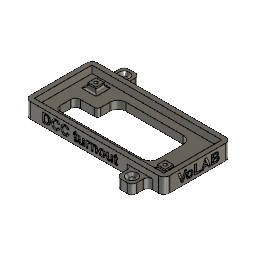
supportCarteDecodeurAiguillage_v4 (Autodesk Fusion 360 design; units mm, degrees)
Autodesk Fusion 360 part; units mm, degrees
note: some values were not read from the file. Chosen so that the rebuilt part matches the saved one: the layout of a text. Set by a fixed rule: which sketch regions a step uses.
sketch "Sketch1" plane through (0, 0, 0) normal (0, 0, 1) x (1, 0, 0)
  line L0 (38.5, -15.24) -> (-38.5, -15.24)
  line L1 (-38.5, -15.24) -> (-38.5, 15.24)
  line L2 (-38.5, 15.24) -> (38.5, 15.24)
  line L3 (38.5, 15.24) -> (38.5, -15.24)
  line L4 (38.5, -15.24) -> (-38.5, 15.24) construction
  line L5 (-38.5, -15.24) -> (38.5, 15.24) construction
  dimension "d1" = 77
  dimension "d2" = 30.48
extrude "Extrude1" add sketch "Sketch1" along normal blind 1.6 makes body 1
sketch "Sketch2" plane through (0, 0, 1.6) normal (0, 0, 1) x (-1, 0, 0)
  line L0 (-38.5, -15.24) -> (38.5, -15.24)
  line L1 (38.5, -15.24) -> (38.5, 15.24)
  line L2 (38.5, 15.24) -> (-38.5, 15.24)
  line L3 (-38.5, 15.24) -> (-38.5, -15.24)
  circle A0 centre (-34.69, 11.43) radius 1.75
  circle A1 centre (31.35, -11.43) radius 1.75
  dimension "d5" = 22.86
  dimension "d6" = 3.5
  dimension "d7" = 3.81
  dimension "d8" = 3.81
  dimension "d9" = 66.04
  dimension "d10" = 4.33
  measures "d6" diameter of A0
extrude "Extrude2" cut sketch "Sketch2" against normal through all contours A0 | A1 bodies 1
copy_body "Body->Comp1" bodies 1 removing the originals makes body 2 in component "carte"
sketch "Sketch3" plane through (0, 0, 0) normal (0, 0, 1) x (1, 0, 0)
  line L0 (43.5, -21) -> (-43.5, -21)
  line L1 (-43.5, -21) -> (-43.5, 21)
  line L2 (-43.5, 21) -> (43.5, 21)
  line L3 (43.5, 21) -> (43.5, -21)
  line L4 (43.5, -21) -> (-43.5, 21) construction
  line L5 (-43.5, -21) -> (43.5, 21) construction
  dimension "d12" = 87
  dimension "d13" = 42
extrude "Extrude3" add sketch "Sketch3" against normal blind 5 from surface at -3 separate body makes body 3
sketch "Sketch4" plane through (0, 0, -3) normal (0, 0, 1) x (-1, 0, 0)
  line L0 (-43.5, -21) -> (43.5, -21)
  line L1 (43.5, -21) -> (43.5, 21)
  line L2 (43.5, 21) -> (-43.5, 21)
  line L3 (-43.5, 21) -> (-43.5, -21)
  circle A0 centre (-34.69, 11.43) radius 1.75
  circle A1 centre (31.35, -11.43) radius 1.75
  line L4 (-37.23, 13.97) -> (-32.15, 13.97)
  line L5 (-32.15, 13.97) -> (-32.15, 8.89)
  line L6 (-32.15, 8.89) -> (-37.23, 8.89)
  line L7 (-37.23, 8.89) -> (-37.23, 13.97)
  line L8 (-37.23, 13.97) -> (-32.15, 8.89) construction
  line L9 (-32.15, 13.97) -> (-37.23, 8.89) construction
  line L10 (28.81, -8.89) -> (33.89, -8.89)
  line L11 (33.89, -8.89) -> (33.89, -13.97)
  line L12 (33.89, -13.97) -> (28.81, -13.97)
  line L13 (28.81, -13.97) -> (28.81, -8.89)
  line L14 (28.81, -8.89) -> (33.89, -13.97) construction
  line L15 (33.89, -8.89) -> (28.81, -13.97) construction
  dimension "d17" = 5.08
  dimension "d18" = 5.08
  dimension "d19" = 5.08
  dimension "d20" = 5.08
extrude "Extrude4" add sketch "Sketch4" along normal blind 3 contours A0 | A1 | L4 L5 L6 L7 | L10 L11 L12 L13 bodies 3
sketch "Sketch5" plane through (0, 0, 0) normal (0, 0, 1) x (-1, 0, 0)
  line L0 (28.81, -13.97) -> (33.89, -13.97)
  line L1 (33.89, -13.97) -> (33.89, -8.89)
  line L2 (33.89, -8.89) -> (28.81, -8.89)
  line L3 (28.81, -8.89) -> (28.81, -13.97)
  line L4 (-32.15, 8.89) -> (-37.23, 13.97) construction
  circle A0 centre (-34.69, 11.43) radius 1
  line L5 (33.89, -13.97) -> (28.81, -8.89) construction
  circle A1 centre (31.35, -11.43) radius 1
  dimension "d25" = 2
  dimension "d26" = 2
  measures "d25" diameter of A0
  measures "d26" diameter of A1
extrude "Extrude6" cut sketch "Sketch5" against normal through all contours A0 | A1 bodies 3
sketch "Sketch6" plane through (0, 0, -3) normal (0, 0, 1) x (-1, 0, 0)
  line L0 (28.81, -13.97) -> (28.81, -8.89)
  line L1 (28.81, -8.89) -> (33.89, -8.89)
  line L2 (33.89, -8.89) -> (33.89, -13.97)
  line L3 (33.89, -13.97) -> (28.81, -13.97)
  line L4 (-37.23, 8.89) -> (-37.23, 13.97)
  line L5 (-37.23, 13.97) -> (-32.15, 13.97)
  line L6 (-32.15, 13.97) -> (-32.15, 8.89)
  line L7 (-32.15, 8.89) -> (-37.23, 8.89)
  line L8 (-43.5, -21) -> (43.5, -21)
  line L9 (43.5, -21) -> (43.5, 21)
  line L10 (43.5, 21) -> (-43.5, 21)
  line L11 (-43.5, 21) -> (-43.5, -21)
  line L12 (-40.5, 18) -> (40.5, 18)
  line L13 (40.5, 18) -> (40.5, -18)
  line L14 (40.5, -18) -> (-40.5, -18)
  line L15 (-40.5, -18) -> (-40.5, 18)
  line L16 (-40.5, 18) -> (40.5, -18) construction
  line L17 (40.5, 18) -> (-40.5, -18) construction
  dimension "d28" = 3
  dimension "d29" = 3
  measures "d28" distance of L8 L14
  measures "d29" distance of L11 L15
extrude "Extrude7" add sketch "Sketch6" along normal blind 4.6 contours L8 L9 L10 L11 bodies 3
fillet "Fillet1" radius 2 8 edges at (-31.35, 8.89, -3) (-28.81, 11.43, -3) (-31.35, 13.97, -3) (-33.89, 11.43, -3) (32.15, -11.43, -3) (34.69, -13.97, -3) (34.69, -8.89, -3) (37.23, -11.43, -3) on bodies 3
fillet "Fillet2" radius 3.5 4 edges at (-43.5, 21, -3.2) (43.5, 21, -3.2) (43.5, -21, -3.2) (-43.5, -21, -3.2) on bodies 3
sketch "Sketch7" plane through (0, 0, -8) normal (0, 0, -1) x (1, 0, 0)
  arc A0 (-40, 21) -> (-43.5, 17.5) centre (-40, 17.5) ccw
  line L0 (-43.5, 17.5) -> (-43.5, -17.5)
  arc A1 (-43.5, -17.5) -> (-40, -21) centre (-40, -17.5) ccw
  line L1 (-40, -21) -> (40, -21)
  arc A2 (40, -21) -> (43.5, -17.5) centre (40, -17.5) ccw
  line L2 (43.5, -17.5) -> (43.5, 17.5)
  arc A3 (43.5, 17.5) -> (40, 21) centre (40, 17.5) ccw
  line L3 (40, 21) -> (-40, 21)
  circle A4 centre (-31.35, -11.43) radius 1
  circle A5 centre (34.69, 11.43) radius 1
  line L4 (33.5, 21) -> (23.5, 21)
  line L5 (23.5, 21) -> (23.5, 31)
  line L6 (23.5, 31) -> (33.5, 31)
  line L7 (33.5, 31) -> (33.5, 21)
  line L8 (-33.5, -21) -> (-23.5, -21)
  line L9 (-23.5, -21) -> (-23.5, -31)
  line L10 (-23.5, -31) -> (-33.5, -31)
  line L11 (-33.5, -31) -> (-33.5, -21)
  line L12 (-33.5, -21) -> (-23.5, -31) construction
  line L13 (23.5, 31) -> (33.5, 21) construction
  circle A6 centre (-28.5, -26) radius 1.8
  circle A7 centre (28.5, 26) radius 1.8
  dimension "d34" = 10
  dimension "d35" = 10
  dimension "d36" = 10
  dimension "d37" = 10
  dimension "d38" = 10
  dimension "d39" = 10
  dimension "d40" = 3.6
  dimension "d41" = 3.6
  measures "d38" distance of L2 L7
  measures "d39" distance of L0 L11
  measures "d40" diameter of A6
  measures "d41" diameter of A7
extrude "Extrude8" add sketch "Sketch7" against normal blind 6 contours L3 L4 L5 L6 L7 | L1 L8 L9 L10 L11 bodies 3
fillet "Fillet3" radius 3 8 edges at (-33.5, 31, -5) (-23.5, 31, -5) (-23.5, 21, -5) (-33.5, 21, -5) (23.5, -31, -5) (23.5, -21, -5) (33.5, -21, -5) (33.5, -31, -5) on bodies 3
chamfer "Chamfer1" distance 1.6 angle 45 2 edges at (26.8218, -25.3491, -2) (-30.1782, 26.6509, -2) on bodies 3
sketch "Sketch8" plane through (0, 0, -3) normal (0, 0, 1) x (-1, 0, 0)
  line L0 (26.81, -15.97) -> (26.81, -6.89)
  line L1 (26.81, -6.89) -> (35.89, -6.89)
  line L2 (35.89, -6.89) -> (35.89, -15.97)
  line L3 (35.89, -15.97) -> (26.81, -15.97)
  line L4 (40.5, -18) -> (40.5, 18)
  line L5 (40.5, 18) -> (-40.5, 18)
  line L6 (-40.5, 18) -> (-40.5, -18)
  line L7 (-40.5, -18) -> (40.5, -18)
  line L8 (-39.23, 6.89) -> (-39.23, 15.97)
  line L9 (-39.23, 15.97) -> (-30.15, 15.97)
  line L10 (-30.15, 15.97) -> (-30.15, 6.89)
  line L11 (-30.15, 6.89) -> (-39.23, 6.89)
  line L12 (14.3781, -13.1158) -> (-21.2623, -13.1158)
  line L13 (-26.2623, -8.1158) -> (-26.2623, 7.3549)
  line L14 (-21.2623, 12.3549) -> (16.3025, 12.3549)
  arc A0 (14.3781, -13.1158) -> (19.3781, -8.1158) centre (14.3781, -8.1158) ccw
  arc A1 (-26.2623, -8.1158) -> (-21.2623, -13.1158) centre (-21.2623, -8.1158) ccw
  arc A2 (-21.2623, 12.3549) -> (-26.2623, 7.3549) centre (-21.2623, 7.3549) ccw
  line L15 (16.3025, 12.3549) -> (30.0989, 12.3549)
  line L16 (33.0989, 9.3549) -> (33.0989, 2.6196)
  line L17 (30.0989, -0.3804) -> (21.3781, -0.3804)
  line L18 (19.3781, -2.3804) -> (19.3781, -8.1158)
  line L19 (9.4549, 12.3549) -> (16.3025, 12.3549)
  arc A3 (30.0989, -0.3804) -> (33.0989, 2.6196) centre (30.0989, 2.6196) ccw
  arc A4 (33.0989, 9.3549) -> (30.0989, 12.3549) centre (30.0989, 9.3549) ccw
  arc A5 (21.3781, -0.3804) -> (19.3781, -2.3804) centre (21.3781, -2.3804) ccw
  dimension "d46" = 5
  dimension "d48" = 3
  dimension "d49" = 2
  measures "d46" radius of A0
  measures "d48" radius of A3
  measures "d49" radius of A5
extrude "Extrude9" cut sketch "Sketch8" against normal through all contours L12 L13 L14 A0 A1 A2 L15 L16 L17 L18 L19 A3 A4 A5 bodies 3
sketch "Sketch9" plane through (43.5, 0, 0) normal (1, 0, 0) x (0, 1, 0)
  line L0 (-17.5, 1.6) -> (-17.5, -8)
  line L1 (-17.5, -8) -> (17.5, -8)
  line L2 (17.5, -8) -> (17.5, 1.6)
  line L3 (17.5, 1.6) -> (-17.5, 1.6)
  line L4 (-12.2296, -6.1338) -> (13.4501, -6.1338) construction
  line L5 (13.4501, -6.1338) -> (13.4501, 1.8662) construction
  line L6 (13.4501, 1.8662) -> (-12.2296, 1.8662) construction
  line L7 (-12.2296, 1.8662) -> (-12.2296, -6.1338) construction
  text T0 "VoLAB" font "Arial" height 8 bold align ink ink in box 0 x 0 at (-12.2196, -6.1138) x (1, 0) y (0, 1) spacing 1 kerned height is em
extrude "Extrude10" cut sketch "Sketch9" against normal blind 2 text T0 bodies 3
sketch "Sketch10" plane through (0, -21, 0) normal (0, -1, 0) x (1, 0, 0)
  line L0 (36.5, -2) -> (36.5, -8)
  line L1 (36.5, -8) -> (40, -8)
  line L2 (40, -8) -> (40, 1.6)
  line L3 (40, 1.6) -> (-40, 1.6)
  line L4 (-40, 1.6) -> (-40, -8)
  line L5 (-40, -8) -> (20.5, -8)
  line L6 (20.5, -8) -> (20.5, -2)
  line L7 (20.5, -2) -> (36.5, -2)
  line L8 (-32.2257, -5.9873) -> (14.6415, -5.9873) construction
  line L9 (14.6415, -5.9873) -> (14.6415, 2.0127) construction
  line L10 (14.6415, 2.0127) -> (-32.2257, 2.0127) construction
  line L11 (-32.2257, 2.0127) -> (-32.2257, -5.9873) construction
  text T0 "DCC turnout" font "Arial" height 8 bold align ink ink in box 0 x 0 at (-32.2157, -5.9673) x (1, 0) y (0, 1) spacing 1 height is em
extrude "Extrude11" cut sketch "Sketch10" against normal blind 2 text T0 bodies 3
component "carte" placed x (1, 0, 0) y (0, 1, 0) z (0, 0, 1) at (0, 0, 0)
equation "d2 = ( 12 * 2.54 ) * 1 mm"
equation "d5 = ( 9 * 2.54 ) * 1 mm"
equation "d7 = ( 1.5 * 2.54 ) * 1 mm"
equation "d8 = ( 1.5 * 2.54 ) * 1 mm"
equation "d9 = ( 26 * 2.54 ) * 1 mm"
equation "d17 = ( 2 * 2.54 ) * 1 mm"
equation "d18 = d17"
equation "d19 = d17"
equation "d20 = d17"
equation "d29 = d28"
equation "d30 = 3 mm + 1.6 mm"
equation "d35 = d34"
equation "d36 = d34"
equation "d37 = d34"
equation "d41 = d40"
